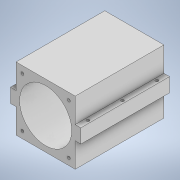
# Autodesk Inventor part: engine_connector_sleeve
Saved by Autodesk Inventor 2020.1 (Build 241239000, 239)
## iProperties
Created: 2022-02-06
Part Number: engine_connector_sleeve
Material: Generic
Document SubType Name: Modeling
Designer: OEM
Density: 1 g/cm^3
Appearance: Default
Author: OEM
Autodesk Inventor part; units mm, degrees
ref_plane "YZ Plane" through (0, 0, 0) normal (1, 0, 0) x (0, 1, 0)
ref_plane "XZ Plane" through (0, 0, 0) normal (0, 1, 0) x (-1, 0, 0)
ref_plane "XY Plane" through (0, 0, 0) normal (0, 0, 1) x (1, 0, 0)
sketch "Sketch1" plane through (0, 0, 0) normal (0, 1, 0) x (-1, 0, 0)
  circle A0 centre (0, 0) radius 11 construction
  circle A1 centre (0, 0) radius 3.75
  circle A2 centre (0, 0) radius 7.875 construction
  line L0 (16.292, 0) -> (-19, 0) construction
  line L1 (0, 21) -> (0, -27.3544) construction
  line L2 (0, -21) -> (21, -21)
  line L3 (0, -21) -> (-21, -21)
  line L4 (0, 0) -> (21, -21) construction
  circle A3 centre (5.5685, -5.5685) radius 0.75
  circle A4 centre (-5.5685, -5.5685) radius 0.75
  circle A5 centre (5.5685, 5.5685) radius 0.75
  circle A6 centre (-5.5685, 5.5685) radius 0.75
  line L5 (-25, -21) -> (-21, -21)
  line L6 (25, -21) -> (21, -21)
  circle A7 centre (23, -14) radius 1
  circle A8 centre (-23, -14) radius 1
  line L7 (-25, 42) -> (25, 42)
  line L8 (25, -21) -> (25, 42)
  line L9 (21, -21) -> (21, 42)
  line L10 (-21, -21) -> (-21, 42)
  line L11 (-25, -21) -> (-25, 42)
  line L12 (25, 10.5) -> (-25, 10.5) construction
  circle A9 centre (23, 35) radius 1
  circle A10 centre (-23, 35) radius 1
  circle A11 centre (23, 10.5) radius 1
  circle A12 centre (-23, 10.5) radius 1
  circle A13 centre (5.5685, 5.5685) radius 1.5
  circle A14 centre (5.5685, -5.5685) radius 1.5
  circle A15 centre (-5.5685, 5.5685) radius 1.5
  circle A16 centre (-5.5685, -5.5685) radius 1.5
  dimension "d8" = 15.75
  dimension "d2" = 7.5
  dimension "d4" = 22
  dimension "d17" = 21
  dimension "d26" = 1.5
  dimension "d38" = 63
  dimension "d39" = 21
  dimension "d40" = 2
  dimension "d41" = 2
  dimension "d53" = 3
  constraints: 26 end point, 16 centre point, 11 symmetric about line, 5 perpendicular, 5 point on line, 2 coincident, 2 midpoint, 1 horizontal, 1 parallel, 1 vertical, 13 other
  measures "d2" diameter of A1
  measures "d4" diameter of A0
  measures "d17" distance from line of point (0, 0) L2
  measures "d26" diameter of A3
  measures "d38" distance of L6.start L7.end
  measures "d39" distance of L2.start L2.end
  measures "d40" diameter of A9
  measures "d41" diameter of A11
  measures "d53" diameter of A13
extrude "Extrusion9" add sketch "Sketch1" along normal blind 45 contours A1 | L3 L10 L7 L9 L2 | A3 | A4 | A5 | A6 | A13 | A14 | A15 | A16
extrude "Extrusion10" add sketch "Sketch1" along normal blind 27.5 contours L9 L7 L8 L6 | L5 L11 L7 L10
extrude "Extrusion11" cut sketch "Sketch1" along normal blind 17.5 contours L9 L7 L8 L6 | L5 L11 L7 L10
extrude "Extrusion13" cut sketch "Sketch1" along normal blind 6 contours A1 | A3 | A4 | A5 | A6 | A13 | A14 | A15 | A16
extrude "Extrusion15" add sketch "Sketch1" along normal blind 3.5 contours A13 | A14 | A15 | A16
sketch "Sketch5" plane through (-21, 45, 42) normal (0, 0, 1) x (1, 0, 0)
  line L0 (0, -45) -> (42, -45) construction
  line L1 (0, -17.5) -> (0, 0) construction
  line L2 (42, -45) -> (0, -45) construction
  line L3 (0, -45) -> (0, 0) construction
  line L4 (0, 0) -> (42, 0) construction
  line L5 (42, 0) -> (42, -45) construction
  line L6 (42, 0) -> (0, -45) construction
  line L7 (0, 0) -> (42, 0) construction
  line L8 (0, 0) -> (42, -45) construction
  circle A0 centre (21, -22.5) radius 18.5
  line L9 (-4, -27.5) -> (-4, -17.5) construction
  line L10 (-4, -22.5) -> (45.9746, -22.5) construction
  line L11 (-4, -23.5) -> (45.9746, -23.5) construction
  line L12 (45.9746, -23.5) -> (45.9746, -45) construction
  line L13 (45.9746, -45) -> (-4, -45) construction
  line L14 (-4, -45) -> (-4, -23.5) construction
  line L15 (-4, -21.5) -> (46, -21.5) construction
  line L16 (46, -21.5) -> (46, 0) construction
  line L17 (46, 0) -> (-4, 0) construction
  line L18 (-4, 0) -> (-4, -21.5) construction
  line L19 (-4, -21.5) -> (45.9746, -21.5) construction
  line L20 (45.9746, -21.5) -> (45.9746, -23.5) construction
  line L21 (45.9746, -23.5) -> (-4, -23.5) construction
  line L22 (-4, -23.5) -> (-4, -21.5) construction
  line L23 (10.2856, -7.4185) -> (31.7144, -7.4185)
  line L24 (5.9185, -11.7856) -> (5.9185, -33.2144)
  line L25 (36.0815, -11.7856) -> (36.0815, -33.2144)
  circle A1 centre (21, -22.5) radius 13.5 construction
  line L26 (21, -22.5) -> (38.8515, -22.5) construction
  line L27 (34.0815, -9.4185) -> (7.9185, -35.5815) construction
  line L28 (21, -45) -> (21, 0) construction
  line L29 (7.9185, -9.4185) -> (34.0815, -35.5815) construction
  line L30 (7.9185, -9.4185) -> (34.0815, -9.4185) construction
  line L31 (7.9185, -9.4185) -> (7.9185, -35.5815) construction
  line L32 (34.0815, -35.5815) -> (34.0815, -9.4185) construction
  circle A2 centre (4.5, -40.1786) radius 1
  circle A3 centre (37.5, -40.1786) radius 1
  circle A4 centre (4.5, -4.8214) radius 1
  circle A5 centre (37.5, -4.8214) radius 1
  dimension "d58" = 37
  dimension "d61" = 1
  dimension "d62" = 1
  dimension "d70" = 27
  dimension "d73" = 2
  dimension "d74" = 45
  dimension "d75" = 2
  dimension "d76" = 2
  dimension "d77" = 42
  dimension "d78" = 45
  dimension "d79" = 2
  dimension "d80" = 4.5
  constraints: 58 end point, 8 parallel, 7 horizontal, 6 perpendicular, 5 centre point, 5 symmetric about line, 3 midpoint, 3 point on line, 1 coincident, 1 vertical, 13 other
  measures "d61" distance between parallel lines of L11 L10
  measures "d62" distance between parallel lines of L10 L15
  measures "d70" diameter of A1
  measures "d73" distance between parallel lines of L32 L25
  measures "d74" angle of L28 L27
  measures "d75" distance between parallel lines of L23 L30
  measures "d76" distance between parallel lines of L31 L24
  measures "d77" distance of L0.start L0.end
  measures "d78" distance of L4.end L0.end
  measures "d79" diameter of A2
  measures "d80" distance from line of L3 A2.centre
extrude "Extrusion16" cut sketch "Sketch5" against normal blind 62 contours L25 A0 L24 L23
extrude "Extrusion18" cut sketch "Sketch5" against normal blind 46 contours A0 L25 | L23 A0 | A0 L24
extrude "Extrusion19" cut sketch "Sketch5" against normal blind 5 contours A2 | A3 | A4 | A5
equation "\"d41\" = d40"
body "Solid2"
